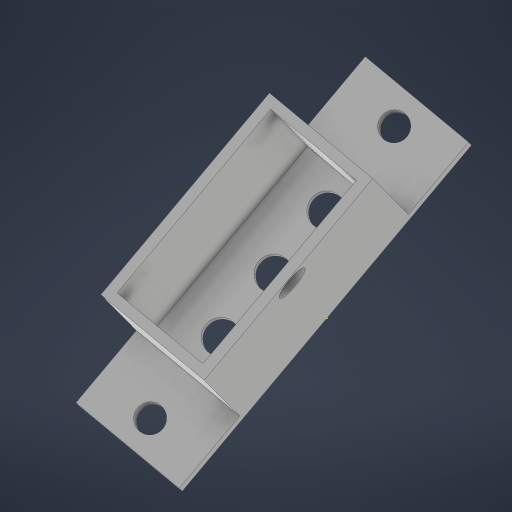
# Autodesk Inventor part: BASE
Saved by Autodesk Inventor 2023 (Build 270158000, 158)
## iProperties
Created: 2023-12-28
Part Number: BASE
Material: Generic
Document SubType Name: Modeling
Designer: User
Density: 1 g/cm^3
Appearance: Default
Author: User
Autodesk Inventor part; units mm, degrees
ref_plane "YZ Plane" through (0, 0, 0) normal (1, 0, 0) x (0, 1, 0)
ref_plane "XZ Plane" through (0, 0, 0) normal (0, 1, 0) x (-1, 0, 0)
ref_plane "XY Plane" through (0, 0, 0) normal (0, 0, 1) x (1, 0, 0)
sketch "Sketch1" plane through (0, 0, 0) normal (0, 0, 1) x (1, 0, 0)
  line L0 (-57.5, 17.5) -> (57.5, 17.5)
  line L1 (57.5, 17.5) -> (57.5, -17.5)
  line L2 (57.5, -17.5) -> (-57.5, -17.5)
  line L3 (-57.5, -17.5) -> (-57.5, 17.5)
  line L4 (-57.5, 17.5) -> (57.5, -17.5) construction
  line L5 (57.5, 17.5) -> (-57.5, -17.5) construction
  point P0 (0, 0)
  dimension "d0" = 115
  dimension "d1" = 35
  constraints: 12 end point, 2 midpoint, 2 parallel, 1 horizontal, 1 perpendicular
  measures "d0" distance of L1.end L2.end
  measures "d1" distance of L0.end L1.end
extrude "Extrusion1" add sketch "Sketch1" along normal blind 5
sketch "Sketch2" plane through (0, 0, 5) normal (0, 0, 1) x (1, 0, 0)
  line L0 (57.5, 17.5) -> (-57.5, 17.5) projected
  line L1 (-33.5, -17.5) -> (33.5, -17.5)
  line L2 (33.5, -17.5) -> (33.5, 17.5)
  line L3 (33.5, 17.5) -> (-33.5, 17.5)
  line L4 (-33.5, 17.5) -> (-33.5, -17.5)
  line L5 (-33.5, -17.5) -> (33.5, 17.5) construction
  line L6 (33.5, -17.5) -> (-33.5, 17.5) construction
  point P0 (0, 0)
  dimension "d10" = 67
  constraints: 12 end point, 2 midpoint, 2 parallel, 1 horizontal, 1 perpendicular, 1 point on line
  measures "d10" distance between parallel lines of L2 L4
extrude "Extrusion2" add sketch "Sketch2" along normal blind 60
shell "Shell1" thickness 3 removed faces 1 at (11.1667, -5.8333, 65)
sketch "Sketch3" plane through (0, 0, 0) normal (0, 0, -1) x (-1, 0, 0)
  circle A0 centre (0, 0) radius 5
  circle A1 centre (21, 0) radius 5
  circle A2 centre (-21, 0) radius 5
  circle A3 centre (48.5, 0) radius 4.25
  circle A4 centre (-48.5, 0) radius 4.25
  line L0 (-57.5, -17.5) -> (-57.5, 17.5) projected
  line L1 (57.5, 17.5) -> (57.5, -17.5) projected
  dimension "d14" = 10
  dimension "d15" = 10
  dimension "d16" = 10
  dimension "d17" = 21
  dimension "d18" = 21
  dimension "d19" = 8.5
  dimension "d20" = 8.5
  dimension "d21" = 97
  dimension "d22" = 9
  dimension "d23" = 9
  constraints: 5 centre point, 3 horizontal alignment, 1 coincident
  measures "d14" diameter of A0
  measures "d15" diameter of A1
  measures "d16" diameter of A2
  measures "d17" distance of A1.centre point (0, 0)
  measures "d18" distance of A2.centre point (0, 0)
  measures "d19" diameter of A3
  measures "d20" diameter of A4
  measures "d21" distance of A4.centre A3.centre
  measures "d22" distance from line of A4.centre L0
  measures "d23" distance from line of L1 A3.centre
extrude "Extrusion3" cut sketch "Sketch3" against normal through all
sketch "Sketch4" plane through (-57.5, -17.5, 0) normal (0, -1, 0) x (1, 0, 0)
  point P0 (57.5, 0)
sketch "Sketch5" plane through (-57.5, -17.5, 0) normal (0, -1, 0) x (1, 0, 0)
  circle A0 centre (57.5, 59) radius 5
  line L0 (24, 65) -> (91, 65) projected
  point P0 (57.5, 0)
  dimension "d26" = 10
  dimension "d27" = 6
  constraints: 1 centre point
  measures "d26" diameter of A0
  measures "d27" distance from line of L0 A0.centre
extrude "Extrusion4" cut sketch "Sketch5" against normal blind 3
body "Solid1"
